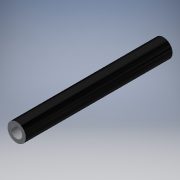
# Autodesk Inventor part: Ellawads thingy
Saved by Autodesk Inventor 2017 (Build 210142000, 142)
## iProperties
Created: 2020-01-14
Part Number: Ellawads thingy
Material: Generic
Document SubType Name: Modeling
Designer: S346553810
Density: 1 g/cm^3
Appearance: Default
Author: S346553810
Autodesk Inventor part; units mm, degrees
ref_plane "YZ Plane" through (0, 0, 0) normal (1, 0, 0) x (0, 1, 0)
ref_plane "XZ Plane" through (0, 0, 0) normal (0, 1, 0) x (-1, 0, 0)
ref_plane "XY Plane" through (0, 0, 0) normal (0, 0, 1) x (1, 0, 0)
sketch "Sketch1" plane through (0, 0, 0) normal (0, 0, 1) x (1, 0, 0)
  circle A0 centre (0.8311, 0.3324) radius 15.875
  point P0 (0, 0)
  dimension "d0" = 31.75
  constraints: 1 centre point
  measures "d0" diameter of A0
extrude "Extrusion1" add sketch "Sketch1" along normal blind 254
sketch "Sketch2" plane through (0.8311, 0.3324, 254) normal (0, 0, 1) x (1, 0, 0)
  circle A0 centre (0, 0) radius 9.525
  point P0 (-0.8311, -0.3324)
  dimension "d3" = 19.05
  constraints: 1 centre point
  measures "d3" diameter of A0
hole "Hole1" at (0.8311, 0.3324, 254) direction (0, 0, -1) diameter 19.05 end through all
body "Solid1"
